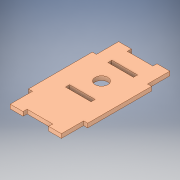
# Autodesk Inventor part: HOMBRO_FONDO
Saved by Autodesk Inventor 2019 (Build 230136000, 136)
## iProperties
Created: 2020-02-12
Part Number: HOMBRO_FONDO
Material: Genérico
Document SubType Name: Modeling
Designer: omar-
Density: 1 g/cm^3
Appearance: Valor por defecto
Author: omar-
Autodesk Inventor part; units mm, degrees
ref_plane "YZ Plane" through (0, 0, 0) normal (1, 0, 0) x (0, 1, 0)
ref_plane "XZ Plane" through (0, 0, 0) normal (0, 1, 0) x (-1, 0, 0)
ref_plane "XY Plane" through (0, 0, 0) normal (0, 0, 1) x (1, 0, 0)
sketch "Boceto1" plane through (0, 0, 0) normal (0, 1, 0) x (-1, 0, 0)
  circle A0 centre (0, 0) radius 5
  line L0 (20, 51.36) -> (-20, 51.36)
  line L1 (-20, 51.36) -> (-20, -33.36)
  line L2 (-20, -33.36) -> (20, -33.36)
  line L3 (20, -33.36) -> (20, 51.36)
  line L4 (10, -15) -> (-10, -15)
  line L5 (-10, -15) -> (-10, -18.18)
  line L6 (-10, -18.18) -> (10, -18.18)
  line L7 (10, -18.18) -> (10, -15)
  line L8 (10, -15) -> (-10, -18.18) construction
  line L9 (-10, -15) -> (10, -18.18) construction
  line L10 (10, -30.18) -> (-10, -30.18)
  line L11 (-10, -30.18) -> (-10, -33.36)
  line L12 (-10, -33.36) -> (10, -33.36)
  line L13 (10, -33.36) -> (10, -30.18)
  line L14 (10, -30.18) -> (-10, -33.36) construction
  line L15 (-10, -30.18) -> (10, -33.36) construction
  line L16 (10, 18.18) -> (-10, 18.18)
  line L17 (-10, 18.18) -> (-10, 15)
  line L18 (-10, 15) -> (10, 15)
  line L19 (10, 15) -> (10, 18.18)
  line L20 (10, 18.18) -> (-10, 15) construction
  line L21 (-10, 18.18) -> (10, 15) construction
  line L22 (10, 51.36) -> (-10, 51.36)
  line L23 (-10, 51.36) -> (-10, 48.18)
  line L24 (-10, 48.18) -> (10, 48.18)
  line L25 (10, 48.18) -> (10, 51.36)
  line L26 (10, 51.36) -> (-10, 48.18) construction
  line L27 (-10, 51.36) -> (10, 48.18) construction
  line L28 (-23.18, 34) -> (-20, 34)
  line L29 (-20, 34) -> (-20, -16)
  line L30 (-20, -16) -> (-23.18, -16)
  line L31 (-23.18, -16) -> (-23.18, 34)
  line L32 (-23.18, 34) -> (-20, -16) construction
  line L33 (-20, 34) -> (-23.18, -16) construction
  line L34 (20, 34) -> (23.18, 34)
  line L35 (23.18, 34) -> (23.18, -16)
  line L36 (23.18, -16) -> (20, -16)
  line L37 (20, -16) -> (20, 34)
  line L38 (20, 34) -> (23.18, -16) construction
  line L39 (23.18, 34) -> (20, -16) construction
  point P0 (0, -16.59)
  point P1 (0, -31.77)
  point P2 (0, 16.59)
  point P3 (0, 49.77)
  point P4 (-21.59, 9)
  point P5 (21.59, 9)
  dimension "d0" = 10
  dimension "d1" = 40
  dimension "d2" = 20
  dimension "d3" = 33.36
  dimension "d5" = 0
  dimension "d6" = 3.18
  dimension "d7" = 20
  dimension "d8" = 3.18
  dimension "d9" = 20
  dimension "d10" = 0
  dimension "d11" = 12
  dimension "d12" = 3.18
  dimension "d13" = 20
  dimension "d14" = 3.18
  dimension "d15" = 20
  dimension "d16" = 0
  dimension "d17" = 0
  dimension "d18" = 30
  dimension "d19" = 30
  dimension "d20" = 3.18
  dimension "d21" = 50
  dimension "d22" = 42.36
  dimension "d23" = 3.18
  dimension "d24" = 50
  dimension "d25" = 42.36
  constraints: 80 end point, 14 parallel, 12 midpoint, 7 horizontal, 7 perpendicular, 4 collinear, 1 centre point, 1 coincident
  measures "d0" diameter of A0
  measures "d1" distance of L1.end L2.end
  measures "d2" distance from line of L3 point (0, 0)
  measures "d3" distance from line of L2 point (0, 0)
  measures "d5" horizontal distance of point (0, 0) point (0, -16.59)
  measures "d6" distance of L6.end L4.start
  measures "d7" distance of L5.end L6.end
  measures "d8" distance of L12.end L10.start
  measures "d9" distance of L11.end L12.end
  measures "d10" horizontal distance of point (0, 0) point (0, -31.77)
  measures "d11" distance between parallel lines of L6 L10
  measures "d12" distance of L19.start L16.start
  measures "d13" distance of L17.end L19.start
  measures "d14" distance of L25.start L22.start
  measures "d15" distance of L23.end L25.start
  measures "d16" horizontal distance of point (0, 0) point (0, 16.59)
  measures "d17" horizontal distance of point (0, 0) point (0, 49.77)
  measures "d18" distance between parallel lines of L18 L4
  measures "d19" distance between parallel lines of L24 L16
  measures "d20" distance of L29.end L30.end
  measures "d21" distance of L28.end L29.end
  measures "d22" distance from line of L2 point (-21.59, 9)
  measures "d23" distance of L38.end L39.end
  measures "d24" distance of L39.start L38.end
  measures "d25" distance from line of L2 point (21.59, 9)
extrude "Extrusión2" add sketch "Boceto1" along normal blind 3.18 contours L3 L2 L13 L10 L11 L1 L0 L23 L24 L25 | L34 L35 L36 L3 | L1 L30 L31 L28
